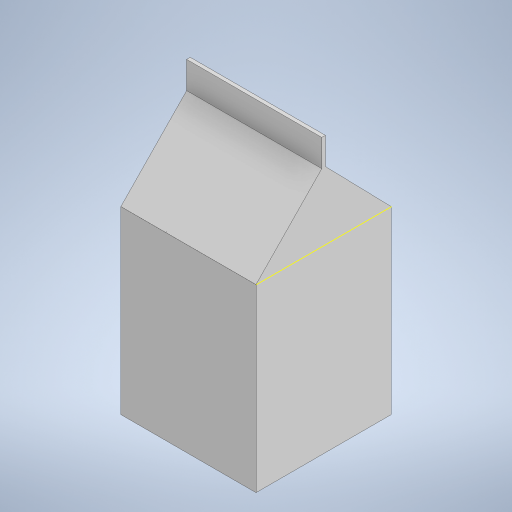
# Autodesk Inventor part: 牛奶瓶
Saved by Autodesk Inventor 2024.2 (Build 282272000, 272)
## iProperties
Created: 2024-03-07
Part Number: 牛奶瓶
Material: 一般
Document SubType Name: Modeling
Designer: User
Density: 1 g/cm^3
Appearance: 預設
Author: User
Autodesk Inventor part; units mm, degrees
ref_plane "YZ Plane" through (0, 0, 0) normal (1, 0, 0) x (0, 1, 0)
ref_plane "XZ Plane" through (0, 0, 0) normal (0, 1, 0) x (-1, 0, 0)
ref_plane "XY Plane" through (0, 0, 0) normal (0, 0, 1) x (1, 0, 0)
sketch "草圖1" plane through (0, 0, 0) normal (0, 0, 1) x (1, 0, 0)
  line L0 (-7.5, 10) -> (7.5, 10)
  line L1 (7.5, 10) -> (7.5, -10)
  line L2 (7.5, -10) -> (-7.5, -10)
  line L3 (-7.5, -10) -> (-7.5, 10)
  line L4 (-7.5, 10) -> (7.5, -10) construction
  line L5 (7.5, 10) -> (-7.5, -10) construction
  point P0 (0, 0)
  dimension "d0" = 15
  dimension "d1" = 20
  constraints: 12 end point, 2 midpoint, 2 parallel, 1 horizontal, 1 perpendicular
  measures "d0" distance of L1.end L2.end
  measures "d1" distance of L0.end L1.end
extrude "擠出1" add sketch "草圖1" along normal blind 15
sketch "草圖2" plane through (-7.5, 10, 0) normal (0, 1, 0) x (1, 0, 0)
  line L0 (0, 0) -> (0, -15) projected
  line L1 (0, -7.5) -> (15, -7.5)
  line L2 (15, 0) -> (15, -15) projected
  point P0 (7.5, 0)
  constraints: 2 end point, 2 midpoint
sketch "草圖3" plane through (7.5, -10, 0) normal (1, 0, 0) x (0, 0, -1)
  line L0 (0, 0) -> (0, 20) projected
  line L1 (0, 20) -> (-15, 20) projected
  line L2 (-15, 0) -> (-15, 20) projected
  line L3 (-15, 20) -> (0, 20)
  line L4 (-7.5, 27.5) -> (-7.3, 27.5)
  line L5 (-7.5, 27.5) -> (-7.7, 27.5)
  line L6 (-7.3, 27.5) -> (0, 20)
  line L7 (-7.7, 27.5) -> (-15.0055, 20)
  line L8 (-7.7, 27.5) -> (-7.7, 30.5)
  line L9 (-7.7, 30.5) -> (-7.3, 30.5)
  line L10 (-7.3, 30.5) -> (-7.3, 27.5)
  line L11 (-15.0055, 20) -> (0, 20)
  point P0 (0, 10)
  point P1 (-7.5, 20)
  dimension "d4" = 7.5
  dimension "d5" = 0.2
  dimension "d6" = 3
  constraints: 18 end point, 2 collinear, 2 perpendicular, 1 horizontal, 1 midpoint, 1 vertical
  measures "d4" distance of point (-7.5, 20) L4.start
  measures "d5" distance of L4.start L4.end
  measures "d6" distance of L5.end L8.end
extrude "擠出3" add sketch "草圖3" against normal blind 15
sketch "草圖4" plane through (-7.5, -10, 0) normal (-1, 0, 0) x (0, 0, 1)
  line L0 (0, 20) -> (7.3, 27.5) projected
  line L1 (0, 20) -> (15.0055, 20)
  line L2 (15.0055, 20) -> (7.5027, 20)
  line L3 (7.3, 30.5) -> (7.3, 27.5) projected
  line L4 (7.5027, 26.3355) -> (0, 20)
  line L5 (7.5027, 26.3355) -> (15.0055, 20)
  point P0 (0, 10)
  constraints: 8 end point, 1 horizontal, 1 midpoint
extrude "擠出4" cut sketch "草圖4" against normal blind 5
